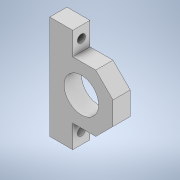
# Autodesk Inventor part: apoyo2
Saved by Autodesk Inventor 2022 (Build 260153000, 153)
## iProperties
Created: 2021-09-11
Part Number: apoyo2
Material: Genérico
Document SubType Name: Modeling
Designer: andre
Density: 1 g/cm^3
Appearance: Valor por defecto
Author: andre
Autodesk Inventor part; units mm, degrees
ref_plane "YZ Plane" through (0, 0, 0) normal (1, 0, 0) x (0, 1, 0)
ref_plane "XZ Plane" through (0, 0, 0) normal (0, 1, 0) x (-1, 0, 0)
ref_plane "XY Plane" through (0, 0, 0) normal (0, 0, 1) x (1, 0, 0)
sketch "Boceto1" plane through (0, 0, 0) normal (0, 0, 1) x (1, 0, 0)
  line L0 (0, 0) -> (20, 0)
  line L1 (20, 0) -> (20, -20)
  line L2 (20, -20) -> (40, -20)
  line L3 (0, 0) -> (0, -90)
  line L4 (0, -90) -> (20, -90)
  line L5 (20, -90) -> (20, -70)
  line L6 (20, -70) -> (40, -70)
  line L7 (40, -20) -> (55, -35)
  line L8 (55, -35) -> (55, -55)
  line L9 (55, -55) -> (40, -70)
  circle A0 centre (27.5, -45) radius 15
  dimension "d0" = 20
  dimension "d1" = 20
  dimension "d2" = 20
  dimension "d3" = 90
  dimension "d4" = 20
  dimension "d5" = 20
  dimension "d6" = 55
  dimension "d7" = 30
  constraints: 20 end point, 5 perpendicular, 2 vertical, 1 centre point, 1 horizontal
  measures "d0" distance of L0.start L0.end
  measures "d1" distance of L0.end L1.end
  measures "d2" distance of L1.end L2.end
  measures "d3" distance of L0.start L3.end
  measures "d4" distance of L4.end L5.end
  measures "d5" distance of L5.end L6.end
  measures "d6" distance between parallel lines of L3 L8
  measures "d7" diameter of A0
extrude "Extrusión1" add sketch "Boceto1" along normal blind 15
sketch "Boceto4" plane through (20, -20, 0) normal (1, 0, 0) x (0, 0, -1)
  line L0 (0, 20) -> (-15, 20) projected
  line L1 (-15, 20) -> (-15, -70) projected
  line L2 (0, 20) -> (0, -70) projected
  circle A0 centre (-7.5, 10) radius 3.5
  line L3 (-15, -70) -> (-15, -50) projected
  line L4 (0, -70) -> (0, -50) projected
  circle A1 centre (-7.5, -60) radius 3.5
  dimension "d19" = 7
  dimension "d20" = 7
  constraints: 2 centre point
  measures "d19" diameter of A0
  measures "d20" diameter of A1
extrude "Extrusión4" cut sketch "Boceto4" against normal blind 20
